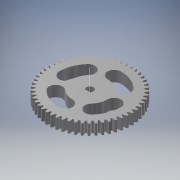
# Autodesk Inventor part: big gear
Saved by Autodesk Inventor 2017 (Build 210142000, 142)
## iProperties
Created: 2018-12-03
Part Number: big gear
Material: Steel
Document SubType Name: Modeling
Designer: Eric the Great
Categories: <?xml version="1.0" encoding="UTF-16"?> <MemberInstance><Categories><FamilyTemplate><FamilyTemplateParameter ValueType="xs:double" Id="1" ObjectReferenceKey="da_z" ObjectType="kUserParameterObject"/><FamilyTemplateParameter ValueType="xs:double" Id="2" ObjectReferenceKey="da_b" ObjectType="kUserParameterObject"/><FamilyTemplateParameter ValueType="xs:double" Id="3" ObjectReferenceKey="da_beta" ObjectType="kUserParameterObject"/><FamilyTemplateParameter ValueType="xs:double" Id="4" ObjectReferenceKey="da_da" ObjectType="kUserParameterObject"/><FamilyTemplateParameter ValueType="xs:double" Id="5" ObjectReferenceKey="da_aw" ObjectType="kUserParameterObject"/><FamilyTemplateParameter ValueType="xs:string" Id="6" ObjectReferenceKey="EAIAABAAAACIAQAAAAAAAIAAAAAAAAAA" ObjectType="83910656" SubObjectId="SurfaceGeometry"/></FamilyTemplate><ParamToTemplateMap><ParamToTemplate CategoryParameter="//CategoryParameter[@InternalName='046C89C9-8512-4d59-83FE-43B91F4F132A']" TemplateParameter="1"/><ParamToTemplate CategoryParameter="//CategoryParameter[@InternalName='2552DF32-E462-4b46-AEBF-C6C7768E72AC']" TemplateParameter="2"/><ParamToTemplate CategoryParameter="//CategoryParameter[@InternalName='C9EE641D-15FC-4fae-A226-E94C4372FDD7']" TemplateParameter="3"/><ParamToTemplate><ParamToTemplate CategoryParameter="//CategoryParameter[@InternalName='00B6519A-459B-49c7-AD84-2E56D39A5744']" ConstantValue="0.344327"/></ParamToTemplate><ParamToTemplate><ParamToTemplate CategoryParameter="//CategoryParameter[@InternalName='04B31F0E-C7A6-4894-AA32-9629BEFACF47']" ConstantValue="1.000000"/></ParamToTemplate><ParamToTemplate><ParamToTemplate CategoryParameter="//CategoryParameter[@InternalName='43CBEC2E-7847-49e7-A936-2F7889FCB2D9']" ConstantValue="0.250000"/></ParamToTemplate><ParamToTemplate><ParamToTemplate CategoryParameter="//CategoryParameter[@InternalName='B1EFC894-105D-4ebd-86BF-FA20ED196853']" ConstantValue="0.350000"/></ParamToTemplate><ParamToTemplate><ParamToTemplate CategoryParameter="//CategoryParameter[@InternalName='51175063-3D10-4879-93E8-6246FE8B403D']" ConstantValue="2060000000.000000"/></ParamToTemplate><ParamToTemplate><ParamToTemplate CategoryParameter="//CategoryParameter[@InternalName='A3A52E27-4454-46a9-B0BD-C932399B70AF']" ConstantValue="0.300000"/></ParamToTemplate><ParamToTemplate><ParamToTemplate CategoryParameter="//CategoryParameter[@InternalName='91B76062-C214-41d9-B1B9-14D2AB99603D']" ConstantValue="0.112500"/></ParamToTemplate><ParamToTemplate><ParamToTemplate CategoryParameter="//CategoryParameter[@InternalName='374E806E-8B8A-4dda-A9AA-1039D6500AD2']" ConstantValue="8.888889"/></ParamToTemplate><ParamToTemplate><ParamToTemplate CategoryParameter="//CategoryParameter[@InternalName='2D373A89-B862-43d6-8D0B-0CBF12AB9F6C']" ConstantValue="0.349066"/></ParamToTemplate><ParamToTemplate CategoryParameter="//CategoryParameter[@InternalName='37777632-D6A2-4fac-9D53-DB8ACD95C989']" TemplateParameter="4"/><ParamToTemplate CategoryParameter="//CategoryParameter[@InternalName='FD1017F1-B727-4f7e-9707-0F86F1FF9423']" TemplateParameter="5"/><ParamToTemplate><ParamToTemplate CategoryParameter="//CategoryParameter[@InternalName='9E1B4470-B2D3-4ff1-B813-535BB4CDF51A']" ConstantValue="3520000.000000"/></ParamToTemplate><ParamToTemplate><ParamToTemplate CategoryParameter="//CategoryParameter[@InternalName='F8452263-BFF6-458c-9FB1-07C4B99E95CD']" ConstantValue="11400000.000000"/></ParamToTemplate><ParamToTemplate><ParamToTemplate CategoryParameter="//CategoryParameter[@InternalName='3E3BB259-FD49-497f-8171-6EBC954A3479']" ConstantValue="2.000000"/></ParamToTemplate><ParamToTemplate CategoryParameter="//CategoryParameter[@InternalName='27C3BAF2-7550-4e4b-AE2C-0DB134B7D9B7']" TemplateParameter="6"/></ParamToTemplateMap><Category DisplayName="Gear" InternalName="DC85795E-93AB-48d5-8EEE-5A27447B64BD" Mnemonic="Gear"><CategoryParameter DisplayName="z" InternalName="046C89C9-8512-4d59-83FE-43B91F4F132A" Mnemonic="z"/><CategoryParameter DisplayName="b" InternalName="2552DF32-E462-4b46-AEBF-C6C7768E72AC" Mnemonic="b"/><CategoryParameter DisplayName="||b|" InternalName="C9EE641D-15FC-4fae-A226-E94C4372FDD7" Mnemonic="beta"/><CategoryParameter DisplayName="x" InternalName="00B6519A-459B-49c7-AD84-2E56D39A5744" Mnemonic="x"/><CategoryParameter DisplayName="a*" InternalName="04B31F0E-C7A6-4894-AA32-9629BEFACF47" Mnemonic="a"/><CategoryParameter DisplayName="c*" InternalName="43CBEC2E-7847-49e7-A936-2F7889FCB2D9" Mnemonic="c"/><CategoryParameter DisplayName="r|.f|*" InternalName="B1EFC894-105D-4ebd-86BF-FA20ED196853" Mnemonic="rf"/><CategoryParameter DisplayName="E" InternalName="51175063-3D10-4879-93E8-6246FE8B403D" Mnemonic="E"/><CategoryParameter DisplayName="||m|" InternalName="A3A52E27-4454-46a9-B0BD-C932399B70AF" Mnemonic="mi"/><Category DisplayName="SpurGear" InternalName="26C5A22E-A91E-4dfd-A3B3-23CCAFAE1764" Mnemonic="SpurGear"><CategoryParameter DisplayName="m" InternalName="91B76062-C214-41d9-B1B9-14D2AB99603D" Mnemonic="m"/><CategoryParameter DisplayName="P" InternalName="374E806E-8B8A-4dda-A9AA-1039D6500AD2" Mnemonic="PP"/><CategoryParameter DisplayName="||a|" InternalName="2D373A89-B862-43d6-8D0B-0CBF12AB9F6C" Mnemonic="alpha"/><CategoryParameter DisplayName="d|.a|" InternalName="37777632-D6A2-4fac-9D53-DB8ACD95C989" Mnemonic="da"/><CategoryParameter DisplayName="a|.w|" InternalName="FD1017F1-B727-4f7e-9707-0F86F1FF9423" Mnemonic="aw"/><CategoryParameter DisplayName="||s||.Flim|" InternalName="9E1B4470-B2D3-4ff1-B813-535BB4CDF51A" Mnemonic="sFlim"/><CategoryParameter DisplayName="||s||.Hlim|" InternalName="F8452263-BFF6-458c-9FB1-07C4B99E95CD" Mnemonic="sHlim"/><CategoryParameter DisplayName="type" InternalName="3E3BB259-FD49-497f-8171-6EBC954A3479" Mnemonic="type"/><CategoryParameter DisplayName="PitchDiameter" InternalName="27C3BAF2-7550-4e4b-AE2C-0DB134B7D9B7" Mnemonic="IDS_PITCHDIAM"/></Category></Category></Categories></MemberInstance>
Density: 1 g/cm^3
Appearance: Steel
CustomPartVersion: 1
Author: Eric the Great
Autodesk Inventor part; units mm, degrees
sketch "Sketch1" plane through (0, 0, 0) normal (0, 0, 1) x (1, 0, 0)
  circle A0 centre (0, 0) radius 31.3125
  dimension "d0" = 62.625
  constraints: 1 centre point
  measures "d0" diameter of A0
extrude "Extrusion1" add sketch "Sketch1" along normal blind 8
ref_plane "Work Plane2" through (0, 0, 4) normal (0, 0, 1) x (1, 0, 0)
sketch "Sketch2" plane through (0, 0, 0) normal (0, 0, -1) x (-1, 0, 0)
  circle A0 centre (0, 0) radius 31.3125 projected
  circle A1 centre (0, 0) radius 30.0811
  dimension "d3" = 60.1622
  constraints: 1 centre point, 1 coincident
  measures "d3" diameter of A1
surface extrude "Pitch Diameter" sketch "Sketch2" against normal through all shown no curves A1
ref_plane "Work Plane8" through (0, 0, 0) normal (0.9982437, 0.0592406, 0) x (0, 0, 1)
ref_plane "Work Plane9" through (0, 0, 0) normal (1, 0, 0) x (0, 1, 0)
spur gear teeth "Spur Gear" teeth 53 pitch diameter 59.625 tip diameter 62.625 root diameter 57.5872 face width 8 start plane through (0, 0, 0) normal (0, 0, -1) x (-1, 0, 0)
sketch "Sketch3" plane through (0, 0, 8) normal (0, 0, 1) x (1, 0, 0)
  circle A0 centre (0, 0) radius 2.65
  line L0 (1.8974, -1.85) -> (-1.8974, -1.85)
  line L1 (0, -1.85) -> (0, 2.65)
  arc A1 (-12.1383, -13.4374) -> (0, -18.1081) centre (0, 0) ccw construction
  arc A2 (-15.4899, -17.1478) -> (0, -23.1081) centre (0, 0) ccw
  arc A3 (-8.7866, -9.7271) -> (0, -13.1081) centre (0, 0) ccw
  arc A4 (-8.7866, -9.7271) -> (-15.4899, -17.1478) centre (-12.1383, -13.4374) ccw
  arc A5 (0, -23.1081) -> (0, -13.1081) centre (0, -18.1081) ccw
  arc A6 (13.4374, -12.1383) -> (18.1081, 0) centre (0, 0) ccw construction
  arc A7 (17.1478, -15.4899) -> (23.1081, 0) centre (0, 0) ccw
  arc A8 (9.7271, -8.7866) -> (13.1081, 0) centre (0, 0) ccw
  arc A9 (9.7271, -8.7866) -> (17.1478, -15.4899) centre (13.4374, -12.1383) ccw
  arc A10 (23.1081, 0) -> (13.1081, 0) centre (18.1081, 0) ccw
  arc A11 (12.1383, 13.4374) -> (0, 18.1081) centre (0, 0) ccw construction
  arc A12 (15.4899, 17.1478) -> (0, 23.1081) centre (0, 0) ccw
  arc A13 (8.7866, 9.7271) -> (0, 13.1081) centre (0, 0) ccw
  arc A14 (8.7866, 9.7271) -> (15.4899, 17.1478) centre (12.1383, 13.4374) ccw
  arc A15 (0, 23.1081) -> (0, 13.1081) centre (0, 18.1081) ccw
  arc A16 (-13.4374, 12.1383) -> (-18.1081, 0) centre (0, 0) ccw construction
  arc A17 (-17.1478, 15.4899) -> (-23.1081, 0) centre (0, 0) ccw
  arc A18 (-9.7271, 8.7866) -> (-13.1081, 0) centre (0, 0) ccw
  arc A19 (-9.7271, 8.7866) -> (-17.1478, 15.4899) centre (-13.4374, 12.1383) ccw
  arc A20 (-23.1081, 0) -> (-13.1081, 0) centre (-18.1081, 0) ccw
  dimension "d51" = 5.3
  dimension "d52" = 4.5
  dimension "d57" = 10
  dimension "d60" = 360
  constraints: 43 point on circle, 21 centre point, 4 end point, 4 tangent, 2 coincident, 1 horizontal, 1 midpoint, 1 vertical, 49 other
  measures "d51" diameter of A0
  measures "d52" distance of L1.start L1.end
  measures "d57" radial gap between concentric circles of A3 A2
extrude "Extrusion2" cut sketch "Sketch3" against normal blind 17 contours A0 L0 L1 | L1 L0 A0 | A4 A3 A5 A2 | A9 A8 A10 A7 | A14 A13 A15 A12 | A19 A18 A20 A17
sketch "Sketch4" plane through (0, 0, 0) normal (0, 0, -1) x (-1, 0, 0)
  circle A0 centre (0, 0) radius 2.65 projected
  circle A1 centre (0, 0) radius 6
  line L0 (1.8974, -1.85) -> (-1.8974, -1.85) projected
  arc A2 (1.8974, -1.85) -> (-1.8974, -1.85) centre (0, 0) ccw projected
  arc A3 (4.6728, 28.4119) -> (4.1638, 31.0344) centre (-8.8256, 27.1525) ccw projected
  arc A4 (4.1638, 31.0344) -> (3.2423, 31.1442) centre (0, 0) ccw projected
  arc A5 (3.2423, 31.1442) -> (2.1315, 28.7146) centre (14.9564, 24.3198) ccw projected
  arc A6 (2.1315, 28.7146) -> (1.2796, 28.7652) centre (0, 0) ccw projected
  arc A7 (1.2796, 28.7652) -> (0.464, 31.3091) centre (-11.975, 25.918) ccw projected
  arc A8 (0.464, 31.3091) -> (-0.464, 31.3091) centre (0, 0) ccw projected
  arc A9 (-0.464, 31.3091) -> (-1.2796, 28.7652) centre (11.975, 25.918) ccw projected
  arc A10 (-1.2796, 28.7652) -> (-2.1315, 28.7146) centre (0, 0) ccw projected
  arc A11 (-2.1315, 28.7146) -> (-3.2423, 31.1442) centre (-14.9564, 24.3198) ccw projected
  arc A12 (-3.2423, 31.1442) -> (-4.1638, 31.0344) centre (0, 0) ccw projected
  arc A13 (-4.1638, 31.0344) -> (-4.6728, 28.4119) centre (8.8256, 27.1525) ccw projected
  arc A14 (-4.6728, 28.4119) -> (-5.5127, 28.261) centre (0, 0) ccw projected
  arc A15 (-5.5127, 28.261) -> (-6.903, 30.5421) centre (-17.7278, 22.3802) ccw projected
  arc A16 (-6.903, 30.5421) -> (-7.8051, 30.3241) centre (0, 0) ccw projected
  arc A17 (-7.8051, 30.3241) -> (-8.0004, 27.6598) centre (5.5522, 28.0057) ccw projected
  arc A18 (-8.0004, 27.6598) -> (-8.8165, 27.4106) centre (0, 0) ccw projected
  arc A19 (-8.8165, 27.4106) -> (-10.4669, 29.5113) centre (-20.2503, 20.1264) ccw projected
  arc A20 (-10.4669, 29.5113) -> (-11.3368, 29.1882) centre (0, 0) ccw projected
  arc A21 (-11.3368, 29.1882) -> (-11.2156, 26.5195) centre (2.2009, 28.4658) ccw projected
  arc A22 (-11.2156, 26.5195) -> (-11.9966, 26.1755) centre (0, 0) ccw projected
  arc A23 (-11.9966, 26.1755) -> (-13.8838, 28.0662) centre (-22.4886, 17.59) ccw projected
  arc A24 (-13.8838, 28.0662) -> (-14.7094, 27.6425) centre (0, 0) ccw projected
  arc A25 (-14.7094, 27.6425) -> (-14.2735, 25.0068) centre (-1.1813, 28.5263) ccw projected
  arc A26 (-14.2735, 25.0068) -> (-15.0082, 24.5729) centre (0, 0) ccw projected
  arc A27 (-15.0082, 24.5729) -> (-17.1059, 26.2271) centre (-24.4112, 14.8068) ccw projected
  arc A28 (-17.1059, 26.2271) -> (-17.8755, 25.7087) centre (0, 0) ccw projected
  arc A29 (-17.8755, 25.7087) -> (-17.1309, 23.1431) centre (-4.5469, 28.1864) ccw projected
  arc A30 (-17.1309, 23.1431) -> (-17.8092, 22.6253) centre (0, 0) ccw projected
  arc A31 (-17.8092, 22.6253) -> (-20.0878, 24.0199) centre (-25.9911, 11.8156) ccw projected
  arc A32 (-20.0878, 24.0199) -> (-20.7907, 23.4141) centre (0, 0) ccw projected
  arc A33 (-20.7907, 23.4141) -> (-19.7479, 20.9546) centre (-7.8486, 27.4508) ccw projected
  arc A34 (-19.7479, 20.9546) -> (-20.3602, 20.3602) centre (0, 0) ccw projected
  arc A35 (-20.3602, 20.3602) -> (-22.7877, 21.4754) centre (-27.2061, 8.6587) ccw projected
  arc A36 (-22.7877, 21.4754) -> (-23.4141, 20.7907) centre (0, 0) ccw projected
  arc A37 (-23.4141, 20.7907) -> (-22.0876, 18.4718) centre (-11.0402, 26.3298) ccw projected
  arc A38 (-22.0876, 18.4718) -> (-22.6253, 17.8092) centre (0, 0) ccw projected
  arc A39 (-22.6253, 17.8092) -> (-25.1677, 18.6295) centre (-28.0393, 5.3801) ccw projected
  arc A40 (-25.1677, 18.6295) -> (-25.7087, 17.8755) centre (0, 0) ccw projected
  arc A41 (-25.7087, 17.8755) -> (-24.1173, 15.7298) centre (-14.0769, 24.8393) ccw projected
  arc A42 (-24.1173, 15.7298) -> (-24.5729, 15.0082) centre (0, 0) ccw projected
  arc A43 (-24.5729, 15.0082) -> (-27.1944, 15.5221) centre (-28.4788, 2.0261) ccw projected
  arc A44 (-27.1944, 15.5221) -> (-27.6425, 14.7094) centre (0, 0) ccw projected
  arc A45 (-27.6425, 14.7094) -> (-25.8085, 12.767) centre (-16.9159, 23) ccw projected
  arc A46 (-25.8085, 12.767) -> (-26.1755, 11.9966) centre (0, 0) ccw projected
  arc A47 (-26.1755, 11.9966) -> (-28.8394, 12.1968) centre (-28.5185, -1.3564) ccw projected
  arc A48 (-28.8394, 12.1968) -> (-29.1882, 11.3368) centre (0, 0) ccw projected
  arc A49 (-29.1882, 11.3368) -> (-27.1373, 9.6249) centre (-19.5174, 20.8379) ccw projected
  arc A50 (-27.1373, 9.6249) -> (-27.4106, 8.8165) centre (0, 0) ccw projected
  arc A51 (-27.4106, 8.8165) -> (-30.0795, 8.7003) centre (-28.1579, -4.7199) ccw projected
  arc A52 (-30.0795, 8.7003) -> (-30.3241, 7.8051) centre (0, 0) ccw projected
  arc A53 (-30.3241, 7.8051) -> (-28.0852, 6.3477) centre (-21.845, 18.3832) ccw projected
  arc A54 (-28.0852, 6.3477) -> (-28.261, 5.5127) centre (0, 0) ccw projected
  arc A55 (-28.261, 5.5127) -> (-30.8974, 5.0816) centre (-27.4021, -8.0171) ccw projected
  arc A56 (-30.8974, 5.0816) -> (-31.0344, 4.1638) centre (0, 0) ccw projected
  arc A57 (-31.0344, 4.1638) -> (-28.6388, 2.9815) centre (-23.8659, 15.6705) ccw projected
  arc A58 (-28.6388, 2.9815) -> (-28.7146, 2.1315) centre (0, 0) ccw projected
  arc A59 (-28.7146, 2.1315) -> (-31.2816, 1.3916) centre (-26.2615, -11.2017) ccw projected
  arc A60 (-31.2816, 1.3916) -> (-31.3091, 0.464) centre (0, 0) ccw projected
  arc A61 (-31.3091, 0.464) -> (-28.7905, -0.4267) centre (-25.5518, 12.7378) ccw projected
  arc A62 (-28.7905, -0.4267) -> (-28.7652, -1.2796) centre (0, 0) ccw projected
  arc A63 (-28.7652, -1.2796) -> (-31.2266, -2.318) centre (-24.7523, -14.2292) ccw projected
  arc A64 (-31.2266, -2.318) -> (-31.1442, -3.2423) centre (0, 0) ccw projected
  arc A65 (-31.1442, -3.2423) -> (-28.5379, -3.8288) centre (-26.879, 9.6263) ccw projected
  arc A66 (-28.5379, -3.8288) -> (-28.4119, -4.6728) centre (0, 0) ccw projected
  arc A67 (-28.4119, -4.6728) -> (-30.7333, -5.9949) centre (-22.8957, -17.0568) ccw projected
  arc A68 (-30.7333, -5.9949) -> (-30.5421, -6.903) centre (0, 0) ccw projected
  arc A69 (-30.5421, -6.903) -> (-27.8848, -7.1772) centre (-27.8289, 6.3797) ccw projected
  arc A70 (-27.8848, -7.1772) -> (-27.6598, -8.0004) centre (0, 0) ccw projected
  arc A71 (-27.6598, -8.0004) -> (-29.8085, -9.5878) centre (-20.7176, -19.645) ccw projected
  arc A72 (-29.8085, -9.5878) -> (-29.5113, -10.4669) centre (0, 0) ccw projected
  arc A73 (-29.5113, -10.4669) -> (-26.8402, -10.4249) centre (-28.3881, 3.0435) ccw projected
  arc A74 (-26.8402, -10.4249) -> (-26.5195, -11.2156) centre (0, 0) ccw projected
  arc A75 (-26.5195, -11.2156) -> (-28.4653, -13.046) centre (-18.2487, -21.9575) ccw projected
  arc A76 (-28.4653, -13.046) -> (-28.0662, -13.8838) centre (0, 0) ccw projected
  arc A77 (-28.0662, -13.8838) -> (-25.4188, -13.5262) centre (-28.5488, -0.3354) ccw projected
  arc A78 (-25.4188, -13.5262) -> (-25.0068, -14.2735) centre (0, 0) ccw projected
  arc A79 (-25.0068, -14.2735) -> (-26.7225, -16.3212) centre (-15.5236, -23.9617) ccw projected
  arc A80 (-26.7225, -16.3212) -> (-26.2271, -17.1059) centre (0, 0) ccw projected
  arc A81 (-26.2271, -17.1059) -> (-23.6406, -16.4376) centre (-28.3088, -3.7096) ccw projected
  arc A82 (-23.6406, -16.4376) -> (-23.1431, -17.1309) centre (0, 0) ccw projected
  arc A83 (-23.1431, -17.1309) -> (-24.6046, -19.3672) centre (-12.5807, -25.6296) ccw projected
  arc A84 (-24.6046, -19.3672) -> (-24.0199, -20.0878) centre (0, 0) ccw projected
  arc A85 (-24.0199, -20.0878) -> (-21.5306, -19.1183) centre (-27.6713, -7.0317) ccw projected
  arc A86 (-21.5306, -19.1183) -> (-20.9546, -19.7479) centre (0, 0) ccw projected
  arc A87 (-20.9546, -19.7479) -> (-22.1413, -22.1413) centre (-9.4611, -26.9376) ccw projected
  arc A88 (-22.1413, -22.1413) -> (-21.4754, -22.7877) centre (0, 0) ccw projected
  arc A89 (-21.4754, -22.7877) -> (-19.1183, -21.5306) centre (-26.6454, -10.2552) ccw projected
  arc A90 (-19.1183, -21.5306) -> (-18.4718, -22.0876) centre (0, 0) ccw projected
  arc A91 (-18.4718, -22.0876) -> (-19.3672, -24.6046) centre (-6.2087, -27.8675) ccw projected
  arc A92 (-19.3672, -24.6046) -> (-18.6295, -25.1677) centre (0, 0) ccw projected
  arc A93 (-18.6295, -25.1677) -> (-16.4376, -23.6406) centre (-25.2455, -13.3346) ccw projected
  arc A94 (-16.4376, -23.6406) -> (-15.7298, -24.1173) centre (0, 0) ccw projected
  arc A95 (-15.7298, -24.1173) -> (-16.3212, -26.7225) centre (-2.8691, -28.4063) ccw projected
  arc A96 (-16.3212, -26.7225) -> (-15.5221, -27.1944) centre (0, 0) ccw projected
  arc A97 (-15.5221, -27.1944) -> (-13.5262, -25.4188) centre (-23.4912, -16.2269) ccw projected
  arc A98 (-13.5262, -25.4188) -> (-12.767, -25.8085) centre (0, 0) ccw projected
  arc A99 (-12.767, -25.8085) -> (-13.046, -28.4653) centre (0.5107, -28.5462) ccw projected
  arc A100 (-13.046, -28.4653) -> (-12.1968, -28.8394) centre (0, 0) ccw projected
  arc A101 (-12.1968, -28.8394) -> (-10.4249, -26.8402) centre (-21.4071, -18.8914) ccw projected
  arc A102 (-10.4249, -26.8402) -> (-9.6249, -27.1373) centre (0, 0) ccw projected
  arc A103 (-9.6249, -27.1373) -> (-9.5878, -29.8085) centre (3.8834, -28.2854) ccw projected
  arc A104 (-9.5878, -29.8085) -> (-8.7003, -30.0795) centre (0, 0) ccw projected
  arc A105 (-8.7003, -30.0795) -> (-7.1772, -27.8848) centre (-19.0225, -21.2907) ccw projected
  arc A106 (-7.1772, -27.8848) -> (-6.3477, -28.0852) centre (0, 0) ccw projected
  arc A107 (-6.3477, -28.0852) -> (-5.9949, -30.7333) centre (7.2016, -27.6276) ccw projected
  arc A108 (-5.9949, -30.7333) -> (-5.0816, -30.8974) centre (0, 0) ccw projected
  arc A109 (-5.0816, -30.8974) -> (-3.8288, -28.5379) centre (-16.3709, -23.3911) ccw projected
  arc A110 (-3.8288, -28.5379) -> (-2.9815, -28.6388) centre (0, 0) ccw projected
  arc A111 (-2.9815, -28.6388) -> (-2.318, -31.2266) centre (10.4186, -26.5819) ccw projected
  arc A112 (-2.318, -31.2266) -> (-1.3916, -31.2816) centre (0, 0) ccw projected
  arc A113 (-1.3916, -31.2816) -> (-0.4267, -28.7905) centre (-13.4894, -25.1631) ccw projected
  arc A114 (-0.4267, -28.7905) -> (0.4267, -28.7905) centre (0, 0) ccw projected
  arc A115 (0.4267, -28.7905) -> (1.3916, -31.2816) centre (13.4894, -25.1631) ccw projected
  arc A116 (1.3916, -31.2816) -> (2.318, -31.2266) centre (0, 0) ccw projected
  arc A117 (2.318, -31.2266) -> (2.9815, -28.6388) centre (-10.4186, -26.5819) ccw projected
  arc A118 (2.9815, -28.6388) -> (3.8288, -28.5379) centre (0, 0) ccw projected
  arc A119 (3.8288, -28.5379) -> (5.0816, -30.8974) centre (16.3709, -23.3911) ccw projected
  arc A120 (5.0816, -30.8974) -> (5.9949, -30.7333) centre (0, 0) ccw projected
  arc A121 (5.9949, -30.7333) -> (6.3477, -28.0852) centre (-7.2016, -27.6276) ccw projected
  arc A122 (6.3477, -28.0852) -> (7.1772, -27.8848) centre (0, 0) ccw projected
  arc A123 (7.1772, -27.8848) -> (8.7003, -30.0795) centre (19.0225, -21.2907) ccw projected
  arc A124 (8.7003, -30.0795) -> (9.5878, -29.8085) centre (0, 0) ccw projected
  arc A125 (9.5878, -29.8085) -> (9.6249, -27.1373) centre (-3.8834, -28.2854) ccw projected
  arc A126 (9.6249, -27.1373) -> (10.4249, -26.8402) centre (0, 0) ccw projected
  arc A127 (10.4249, -26.8402) -> (12.1968, -28.8394) centre (21.4071, -18.8914) ccw projected
  arc A128 (12.1968, -28.8394) -> (13.046, -28.4653) centre (0, 0) ccw projected
  arc A129 (13.046, -28.4653) -> (12.767, -25.8085) centre (-0.5107, -28.5462) ccw projected
  arc A130 (12.767, -25.8085) -> (13.5262, -25.4188) centre (0, 0) ccw projected
  arc A131 (13.5262, -25.4188) -> (15.5221, -27.1944) centre (23.4912, -16.2269) ccw projected
  arc A132 (15.5221, -27.1944) -> (16.3212, -26.7225) centre (0, 0) ccw projected
  arc A133 (16.3212, -26.7225) -> (15.7298, -24.1173) centre (2.8691, -28.4063) ccw projected
  arc A134 (15.7298, -24.1173) -> (16.4376, -23.6406) centre (0, 0) ccw projected
  arc A135 (16.4376, -23.6406) -> (18.6295, -25.1677) centre (25.2455, -13.3346) ccw projected
  arc A136 (18.6295, -25.1677) -> (19.3672, -24.6046) centre (0, 0) ccw projected
  arc A137 (19.3672, -24.6046) -> (18.4718, -22.0876) centre (6.2087, -27.8675) ccw projected
  arc A138 (18.4718, -22.0876) -> (19.1183, -21.5306) centre (0, 0) ccw projected
  arc A139 (19.1183, -21.5306) -> (21.4754, -22.7877) centre (26.6454, -10.2552) ccw projected
  arc A140 (21.4754, -22.7877) -> (22.1413, -22.1413) centre (0, 0) ccw projected
  arc A141 (22.1413, -22.1413) -> (20.9546, -19.7479) centre (9.4611, -26.9376) ccw projected
  arc A142 (20.9546, -19.7479) -> (21.5306, -19.1183) centre (0, 0) ccw projected
  arc A143 (21.5306, -19.1183) -> (24.0199, -20.0878) centre (27.6713, -7.0317) ccw projected
  arc A144 (24.0199, -20.0878) -> (24.6046, -19.3672) centre (0, 0) ccw projected
  arc A145 (24.6046, -19.3672) -> (23.1431, -17.1309) centre (12.5807, -25.6296) ccw projected
  arc A146 (23.1431, -17.1309) -> (23.6406, -16.4376) centre (0, 0) ccw projected
  arc A147 (23.6406, -16.4376) -> (26.2271, -17.1059) centre (28.3088, -3.7096) ccw projected
  arc A148 (26.2271, -17.1059) -> (26.7225, -16.3212) centre (0, 0) ccw projected
  arc A149 (26.7225, -16.3212) -> (25.0068, -14.2735) centre (15.5236, -23.9617) ccw projected
  arc A150 (25.0068, -14.2735) -> (25.4188, -13.5262) centre (0, 0) ccw projected
  arc A151 (25.4188, -13.5262) -> (28.0662, -13.8838) centre (28.5488, -0.3354) ccw projected
  arc A152 (28.0662, -13.8838) -> (28.4653, -13.046) centre (0, 0) ccw projected
  arc A153 (28.4653, -13.046) -> (26.5195, -11.2156) centre (18.2487, -21.9575) ccw projected
  arc A154 (26.5195, -11.2156) -> (26.8402, -10.4249) centre (0, 0) ccw projected
  arc A155 (26.8402, -10.4249) -> (29.5113, -10.4669) centre (28.3881, 3.0435) ccw projected
  arc A156 (29.5113, -10.4669) -> (29.8085, -9.5878) centre (0, 0) ccw projected
  arc A157 (29.8085, -9.5878) -> (27.6598, -8.0004) centre (20.7176, -19.645) ccw projected
  arc A158 (27.6598, -8.0004) -> (27.8848, -7.1772) centre (0, 0) ccw projected
  arc A159 (27.8848, -7.1772) -> (30.5421, -6.903) centre (27.8289, 6.3797) ccw projected
  arc A160 (30.5421, -6.903) -> (30.7333, -5.9949) centre (0, 0) ccw projected
  arc A161 (30.7333, -5.9949) -> (28.4119, -4.6728) centre (22.8957, -17.0568) ccw projected
  arc A162 (28.4119, -4.6728) -> (28.5379, -3.8288) centre (0, 0) ccw projected
  arc A163 (28.5379, -3.8288) -> (31.1442, -3.2423) centre (26.879, 9.6263) ccw projected
  arc A164 (31.1442, -3.2423) -> (31.2266, -2.318) centre (0, 0) ccw projected
  arc A165 (31.2266, -2.318) -> (28.7652, -1.2796) centre (24.7523, -14.2292) ccw projected
  arc A166 (28.7652, -1.2796) -> (28.7905, -0.4267) centre (0, 0) ccw projected
  arc A167 (28.7905, -0.4267) -> (31.3091, 0.464) centre (25.5518, 12.7378) ccw projected
  arc A168 (31.3091, 0.464) -> (31.2816, 1.3916) centre (0, 0) ccw projected
  arc A169 (31.2816, 1.3916) -> (28.7146, 2.1315) centre (26.2615, -11.2017) ccw projected
  arc A170 (28.7146, 2.1315) -> (28.6388, 2.9815) centre (0, 0) ccw projected
  arc A171 (28.6388, 2.9815) -> (31.0344, 4.1638) centre (23.8659, 15.6705) ccw projected
  arc A172 (31.0344, 4.1638) -> (30.8974, 5.0816) centre (0, 0) ccw projected
  arc A173 (30.8974, 5.0816) -> (28.261, 5.5127) centre (27.4021, -8.0171) ccw projected
  arc A174 (28.261, 5.5127) -> (28.0852, 6.3477) centre (0, 0) ccw projected
  arc A175 (28.0852, 6.3477) -> (30.3241, 7.8051) centre (21.845, 18.3832) ccw projected
  arc A176 (30.3241, 7.8051) -> (30.0795, 8.7003) centre (0, 0) ccw projected
  arc A177 (30.0795, 8.7003) -> (27.4106, 8.8165) centre (28.1579, -4.7199) ccw projected
  arc A178 (27.4106, 8.8165) -> (27.1373, 9.6249) centre (0, 0) ccw projected
  arc A179 (27.1373, 9.6249) -> (29.1882, 11.3368) centre (19.5174, 20.8379) ccw projected
  arc A180 (29.1882, 11.3368) -> (28.8394, 12.1968) centre (0, 0) ccw projected
  arc A181 (28.8394, 12.1968) -> (26.1755, 11.9966) centre (28.5185, -1.3564) ccw projected
  arc A182 (26.1755, 11.9966) -> (25.8085, 12.767) centre (0, 0) ccw projected
  arc A183 (25.8085, 12.767) -> (27.6425, 14.7094) centre (16.9159, 23) ccw projected
  arc A184 (27.6425, 14.7094) -> (27.1944, 15.5221) centre (0, 0) ccw projected
  arc A185 (27.1944, 15.5221) -> (24.5729, 15.0082) centre (28.4788, 2.0261) ccw projected
  arc A186 (24.5729, 15.0082) -> (24.1173, 15.7298) centre (0, 0) ccw projected
  arc A187 (24.1173, 15.7298) -> (25.7087, 17.8755) centre (14.0769, 24.8393) ccw projected
  arc A188 (25.7087, 17.8755) -> (25.1677, 18.6295) centre (0, 0) ccw projected
  arc A189 (25.1677, 18.6295) -> (22.6253, 17.8092) centre (28.0393, 5.3801) ccw projected
  arc A190 (22.6253, 17.8092) -> (22.0876, 18.4718) centre (0, 0) ccw projected
  arc A191 (22.0876, 18.4718) -> (23.4141, 20.7907) centre (11.0402, 26.3298) ccw projected
  arc A192 (23.4141, 20.7907) -> (22.7877, 21.4754) centre (0, 0) ccw projected
  arc A193 (22.7877, 21.4754) -> (20.3602, 20.3602) centre (27.2061, 8.6587) ccw projected
  arc A194 (20.3602, 20.3602) -> (19.7479, 20.9546) centre (0, 0) ccw projected
  arc A195 (19.7479, 20.9546) -> (20.7907, 23.4141) centre (7.8486, 27.4508) ccw projected
  arc A196 (20.7907, 23.4141) -> (20.0878, 24.0199) centre (0, 0) ccw projected
  arc A197 (20.0878, 24.0199) -> (17.8092, 22.6253) centre (25.9911, 11.8156) ccw projected
  arc A198 (17.8092, 22.6253) -> (17.1309, 23.1431) centre (0, 0) ccw projected
  arc A199 (17.1309, 23.1431) -> (17.8755, 25.7087) centre (4.5469, 28.1864) ccw projected
  arc A200 (17.8755, 25.7087) -> (17.1059, 26.2271) centre (0, 0) ccw projected
  arc A201 (17.1059, 26.2271) -> (15.0082, 24.5729) centre (24.4112, 14.8068) ccw projected
  arc A202 (15.0082, 24.5729) -> (14.2735, 25.0068) centre (0, 0) ccw projected
  arc A203 (14.2735, 25.0068) -> (14.7094, 27.6425) centre (1.1813, 28.5263) ccw projected
  arc A204 (14.7094, 27.6425) -> (13.8838, 28.0662) centre (0, 0) ccw projected
  arc A205 (13.8838, 28.0662) -> (11.9966, 26.1755) centre (22.4886, 17.59) ccw projected
  arc A206 (11.9966, 26.1755) -> (11.2156, 26.5195) centre (0, 0) ccw projected
  arc A207 (11.2156, 26.5195) -> (11.3368, 29.1882) centre (-2.2009, 28.4658) ccw projected
  arc A208 (11.3368, 29.1882) -> (10.4669, 29.5113) centre (0, 0) ccw projected
  arc A209 (10.4669, 29.5113) -> (8.8165, 27.4106) centre (20.2503, 20.1264) ccw projected
  arc A210 (8.8165, 27.4106) -> (8.0004, 27.6598) centre (0, 0) ccw projected
  arc A211 (8.0004, 27.6598) -> (7.8051, 30.3241) centre (-5.5522, 28.0057) ccw projected
  arc A212 (7.8051, 30.3241) -> (6.903, 30.5421) centre (0, 0) ccw projected
  arc A213 (6.903, 30.5421) -> (5.5127, 28.261) centre (17.7278, 22.3802) ccw projected
  arc A214 (5.5127, 28.261) -> (4.6728, 28.4119) centre (0, 0) ccw projected
  dimension "d53" = 12
  constraints: 1 centre point, 1 coincident
  measures "d53" diameter of A1
extrude "Extrusion3" add sketch "Sketch4" along normal blind 7 contours L0 A0 | A1 picked at (0.4767, -1.977)
fillet "Fillet1" radius 2 1 edges at (6, 0, 0)
equation "\"d0\" = da_da"
equation "\"d1\" = da_b"
equation "\"d3\" = da_dw"
equation "\"d16\" = da_aw"
equation "\"d43\" = da_aw"
equation "\"d46\" = da_aw"
equation "\"da_da\" = 62.625"
equation "\"da_b\" = 8"
equation "\"da_dw\" = 60.162162"
equation "\"da_aw\" = 42"
body "Solid1"
body "Srf1"
